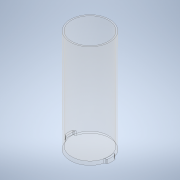
# Autodesk Inventor part: HSI
Saved by Autodesk Inventor 2022 (Build 260153000, 153)
## iProperties
Created: 2022-03-30
Part Number: HSI
Material: Polycarbonate, Clear
Document SubType Name: Modeling
Designer: RNG3nius
Density: 1.2 g/cm^3
Appearance: Polycarbonate - Clear
Author: RNG3nius
Autodesk Inventor part; units mm, degrees
ref_plane "YZ Plane" through (0, 0, 0) normal (1, 0, 0) x (0, 1, 0)
ref_plane "XZ Plane" through (0, 0, 0) normal (0, 1, 0) x (-1, 0, 0)
ref_plane "XY Plane" through (0, 0, 0) normal (0, 0, 1) x (1, 0, 0)
sketch "Sketch1" plane through (0, 0, 0) normal (0, 1, 0) x (-1, 0, 0)
  circle A0 centre (0, 0) radius 28.8
  dimension "d0" = 57.6
  constraints: 1 centre point, 1 coincident
  measures "d0" diameter of A0
extrude "Extrusion1" add sketch "Sketch1" along normal blind 150
sketch "Sketch2" plane through (0, 150, 0) normal (0, 1, 0) x (1, 0, 0)
  point P0 (0, 0)
  point P1 (0, 0)
  constraints: 1 coincident
hole "Hole1" at (0, 150, 0) direction (0, -1, 0) diameter 53.6 depth 146
sketch "Sketch3" plane through (0, 0, 0) normal (0, -1, 0) x (1, 0, 0)
  circle A0 centre (0, 0) radius 31.65
  circle A1 centre (0, 0) radius 28.8 projected
  line L0 (28.0984, -6.3183) -> (28.0984, 6.3183)
  line L1 (28.0984, 6.3183) -> (31.0129, 6.3183)
  line L2 (28.0984, -6.3183) -> (31.0129, -6.3183)
  line L3 (-28.0984, 6.3183) -> (-28.0984, -6.3183)
  line L4 (-28.0984, 6.3183) -> (-31.0129, 6.3183)
  line L5 (-28.0984, -6.3183) -> (-31.0129, -6.3183)
  dimension "d10" = 63.3
  dimension "d13" = 360
  constraints: 12 end point, 5 point on circle, 2 point on line, 1 centre point, 1 coincident, 1 parallel, 1 perpendicular, 1 vertical, 17 other
  measures "d10" diameter of A0
extrude "Extrusion2" add sketch "Sketch3" against normal blind 5.8 contours A0 L2 A1 L1 | L4 A1 L5 A0
fillet "Fillet1" radius 1.4575 8 edges at (28.0984, 2.9, -6.3183) (31.0129, 2.9, -6.3183) (31.0129, 2.9, 6.3183) (28.0984, 2.9, 6.3183) (-31.0129, 2.9, 6.3183) (-28.0984, 2.9, 6.3183) (-31.0129, 2.9, -6.3183) (-28.0984, 2.9, -6.3183)
body "Solid1"
